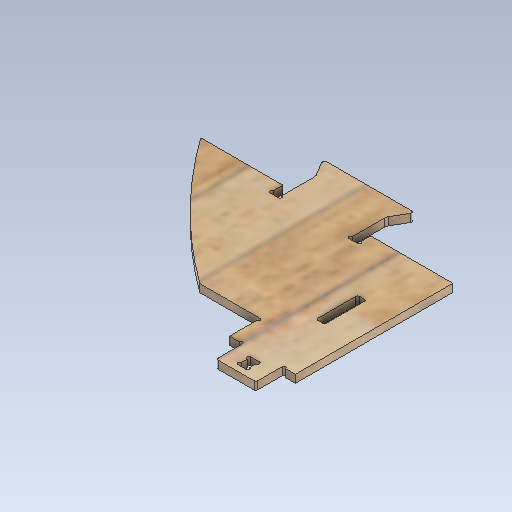
# Autodesk Inventor part: Support A
Saved by Autodesk Inventor 2020 (Build 240168000, 168)
## iProperties
Created: 2020-03-07
Part Number: Support A
Material: Wood (Maple)
Document SubType Name: Modeling
Designer: Daniel Wikman
Density: 0.67 g/cm^3
Appearance: Natural Maple - Glossy Dark Tint
Author: Daniel Wikman
Autodesk Inventor part; units mm, degrees
ref_plane "YZ Plane" through (0, 0, 0) normal (1, 0, 0) x (0, 1, 0)
ref_plane "XZ Plane" through (0, 0, 0) normal (0, 1, 0) x (-1, 0, 0)
ref_plane "XY Plane" through (0, 0, 0) normal (0, 0, 1) x (1, 0, 0)
sketch "Sketch1" plane through (0, 0, 0) normal (0, 1, 0) x (-1, 0, 0)
  line L0 (27.2237, 3.0303) -> (-0.1096, 3.0303)
  line L1 (-1.4429, 1.697) -> (-1.4429, -16.9697)
  arc A0 (-4.1096, -16.9697) -> (-1.4429, -16.9697) centre (-2.7763, -16.9697) ccw
  line L2 (28.5571, 1.697) -> (28.5571, -16.9697)
  arc A1 (28.5571, -16.9697) -> (31.2237, -16.9697) centre (29.8904, -16.9697) ccw
  line L3 (31.2237, -16.9697) -> (38.5571, -16.9697)
  line L4 (-4.1096, -16.9697) -> (-11.4429, -16.9697)
  arc A2 (28.5571, 1.697) -> (27.2237, 3.0303) centre (27.2237, 1.697) ccw
  arc A3 (-0.1096, 3.0303) -> (-1.4429, 1.697) centre (-0.1096, 1.697) ccw
  line L5 (-11.4429, -16.9697) -> (-11.4429, -136.4697)
  line L6 (38.5571, -16.9697) -> (38.5571, -37.6364)
  arc A4 (38.5571, -37.6364) -> (38.5571, -40.303) centre (38.5571, -38.9697) ccw
  line L7 (38.5571, -40.303) -> (84.3904, -40.303)
  line L8 (-11.4429, -136.4697) -> (50.8904, -136.4697)
  line L9 (50.8904, -136.4697) -> (50.8904, -129.1364)
  arc A5 (50.8904, -126.4697) -> (50.8904, -129.1364) centre (50.8904, -127.803) ccw
  arc A6 (57.3904, -129.1364) -> (57.3904, -126.4697) centre (57.3904, -127.803) ccw
  line L10 (57.3904, -126.4697) -> (50.8904, -126.4697)
  arc A7 (50.5474, -166.5079) -> (51.7021, -168.5079) centre (51.7021, -167.1746) ccw
  line L11 (51.7021, -168.5079) -> (116.7021, -168.5079)
  line L12 (84.2021, -168.5079) -> (84.2021, -124.5465)
  line L13 (179.8472, -136.4697) -> (117.5139, -136.4697)
  line L14 (117.5139, -136.4697) -> (117.5139, -129.1364)
  line L15 (111.0139, -153.3159) -> (111.0139, -129.1364)
  arc A8 (117.5139, -129.1364) -> (117.5139, -126.4697) centre (117.5139, -127.803) ccw
  arc A9 (111.0139, -126.4697) -> (111.0139, -129.1364) centre (111.0139, -127.803) ccw
  line L16 (111.0139, -126.4697) -> (117.5139, -126.4697)
  arc A10 (116.7021, -168.5079) -> (117.8568, -166.5079) centre (116.7021, -167.1746) ccw
  arc A11 (179.8472, -136.4697) -> (84.3904, -40.303) centre (-165.6556, -383.9628) ccw
  line L17 (13.5571, -92.4697) -> (11.6404, -92.4697)
  arc A12 (11.6404, -60.9697) -> (10.3071, -62.303) centre (11.6404, -62.303) ccw
  arc A13 (10.3071, -91.1364) -> (11.6404, -92.4697) centre (11.6404, -91.1364) ccw
  arc A14 (16.8071, -11.4697) -> (16.8071, -8.803) centre (16.8071, -10.1364) ccw
  arc A15 (16.8071, -4.1364) -> (16.8071, -1.4697) centre (16.8071, -2.803) ccw
  line L18 (16.8071, -8.803) -> (16.8071, -4.1364)
  line L19 (16.8071, -11.4697) -> (13.5571, -11.4697)
  line L20 (16.8071, -1.4697) -> (13.5571, -1.4697)
  arc A16 (10.3071, -8.803) -> (10.3071, -11.4697) centre (10.3071, -10.1364) ccw
  arc A17 (10.3071, -1.4697) -> (10.3071, -4.1364) centre (10.3071, -2.803) ccw
  line L21 (10.3071, -8.803) -> (10.3071, -4.1364)
  line L22 (10.3071, -11.4697) -> (13.5571, -11.4697)
  line L23 (10.3071, -1.4697) -> (13.5571, -1.4697)
  line L24 (10.3071, -91.1364) -> (10.3071, -62.303)
  line L25 (11.6404, -60.9697) -> (13.5571, -60.9697)
  line L26 (13.5571, -92.4697) -> (15.4737, -92.4697)
  arc A18 (16.8071, -62.303) -> (15.4737, -60.9697) centre (15.4737, -62.303) ccw
  arc A19 (15.4737, -92.4697) -> (16.8071, -91.1364) centre (15.4737, -91.1364) ccw
  line L27 (16.8071, -91.1364) -> (16.8071, -62.303)
  line L28 (15.4737, -60.9697) -> (13.5571, -60.9697)
  line L29 (117.8568, -166.5079) -> (111.6838, -155.8159)
  arc A20 (111.0139, -153.3159) -> (111.6838, -155.8159) centre (116.0139, -153.3159) ccw
  line L30 (57.3904, -153.3159) -> (57.3904, -129.1364)
  line L31 (50.5474, -166.5079) -> (56.7205, -155.8159)
  arc A21 (56.7205, -155.8159) -> (57.3904, -153.3159) centre (52.3904, -153.3159) ccw
  line L32 (13.5571, 3.0303) -> (13.5571, 6.6186)
  point P0 (0, 0)
  point P1 (28.5571, 3.0303)
  point P2 (-1.4429, 3.0303)
  point P3 (111.0139, -159.1364)
  point P4 (12.6821, -76.7197)
  dimension "d1" = 2.6667
  dimension "d2" = 30
  dimension "d3" = 20
  dimension "d4" = 2.6667
  dimension "d5" = 1.3333
  dimension "d6" = 7.3333
  dimension "d7" = 7.3333
  dimension "d8" = 20.6667
  dimension "d9" = 2.6667
  dimension "d10" = 45.8333
  dimension "d11" = 119.5
  dimension "d12" = 62.3333
  dimension "d17" = 2.6667
  dimension "d18" = 2.6667
  dimension "d19" = 7.3333
  dimension "d25" = 2.6667
  dimension "d26" = 65
  dimension "d27" = 425
  dimension "d39" = 44
  dimension "d53" = 2.6667
  dimension "d56" = 2.6667
  dimension "d57" = 4.5
  dimension "d58" = 5.5
  dimension "d59" = 6.5
  dimension "d63" = 1.3333
  dimension "d66" = 44
  dimension "d70" = 191.2902
  dimension "d71" = 62.3333
  dimension "d72" = 67.6667
  dimension "d73" = 9.3716
  dimension "d75" = 32.0382
  dimension "d76" = 60
  dimension "d79" = 5
  dimension "d80" = 70.6451
  constraints: 66 end point, 44 point on circle, 22 centre point, 14 tangent, 13 symmetric about line, 9 horizontal, 8 vertical, 4 point on line, 2 equal radius, 2 midpoint, 1 perpendicular, 4 other
  measures "d1" diameter of A0
  measures "d2" distance of point (28.557, 3.03) point (-1.443, 3.03)
  measures "d3" distance of point (-1.443, 3.03) L1.end
  measures "d4" diameter of A1
  measures "d5" radius of A2
  measures "d6" distance of L3.start L3.end
  measures "d7" distance of L4.start L4.end
  measures "d8" distance of L3.end L6.end
  measures "d9" diameter of A4
  measures "d10" distance of L7.start L7.end
  measures "d11" distance of L4.end L5.end
  measures "d12" distance of L5.end L8.end
  measures "d17" diameter of A5
  measures "d18" diameter of A6
  measures "d19" distance of L8.end L9.end
  measures "d25" diameter of A7
  measures "d26" distance of L11.start L11.end
  measures "d27" radius of A11
  measures "d39" distance between parallel lines of L8 L17
  measures "d53" diameter of A14
  measures "d56" diameter of A15
  measures "d57" distance edge to line of A15 L0
  measures "d58" distance edge to line of A14 L3
  measures "d59" distance between parallel lines of L21 L18
  measures "d63" radius of A13
  measures "d66" distance from line of L25.start L4
  measures "d70" distance of L5.end L13.start
  measures "d71" distance of L13.start L14.start
  measures "d73" distance from line of point (111.014, -159.136) L11
  measures "d75" distance between parallel lines of L8 L11
  measures "d76" angle of L11 L29
  measures "d79" radius of A20
  measures "d80" distance between parallel lines of L12 L32
extrude "Extrusion2" add sketch "Sketch1" along normal blind 6
body "Solid2"
